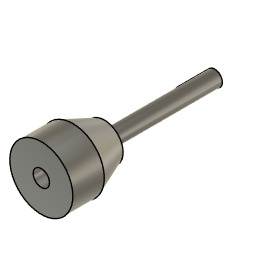
Motor_wheel_holder (Autodesk Fusion 360 archive; units mm, degrees)
design "Shaft"
Autodesk Fusion 360 part; units mm, degrees
sketch "Sketch1" plane through (0, 0, 0) normal (1, 0, 0) x (0, 1, 0)
  line L0 (0, 0) -> (55, 0) construction
  line L1 (55, 0) -> (55, 2.45)
  line L2 (20, 2.45) -> (20, 5.95)
  line L3 (12, 0) -> (9.8183, 2.6)
  line L4 (9.8183, 2.6) -> (0, 2.6)
  line L5 (12, 0) -> (55, 0)
  line L6 (0, 10) -> (0, 2.6)
  line L7 (20, 2.45) -> (55, 2.45)
  line L8 (0, 10) -> (10, 9.9769)
  line L9 (10, 9.9769) -> (20, 5.95)
  dimension "d1" = 2.45
  dimension "d3" = 50
  dimension "d4" = 12
  dimension "d5" = 20
  dimension "d7" = 2.6
  dimension "d8" = 55
  dimension "d18" = 10
  dimension "d19" = 10
  dimension "d20" = 158.199
  dimension "d21" = 3.5
  constraint coincident L0.start origin
  constraint horizontal L0
  constraint perpendicular L0 L1
  constraint coincident L0 L3.start
  constraint parallel L0 L4
  constraint perpendicular L4 L6
  constraint coincident L0.start L6
  constraint perpendicular L1 L7
  measures "d1" distance of L0.end L1.end
  measures "d3" angle of L0 L3
  measures "d4" distance of L3.start L6
  measures "d5" distance of L2 L6
  measures "d7" distance of L0.start L4
  measures "d8" distance of L1 L4.end
  measures "d18" distance of L0.start L8
  measures "d19" distance of L8.end L6.start
  measures "d20" angle of L8 L9
  measures "d21" distance of L2.end L7
revolve "Revolve1" add sketch "Sketch1" angle 360 about axis through (0, 0, 0) along (0, 1, 0)
ref_plane "WorkPlane1" through (-2.45, 48.8519, 0) normal (-1, 0, 0) x (0, 0, -1)
sketch "Sketch2" plane through (-2.45, 0, 0) normal (-1, 0, 0) x (0, -1, 0)
  line L0 (-55, -5) -> (-45, -5)
  line L1 (-45, -5) -> (-45, 5)
  line L2 (-45, 5) -> (-55, 5)
  line L3 (-55, 5) -> (-55, -5)
  constraint horizontal L0
  constraint vertical L1
  constraint horizontal L2
  constraint vertical L3
extrude "Extrude1" cut sketch "Sketch2" against normal blind 0.5
ref_plane "WorkPlane2" through (-9.9885, 5, 0) normal (-0.999997, 0.002314, 0) x (0, 0, -1)
sketch "Sketch3" plane through (-10, 0.0231, 0) normal (-0.999997, 0.002314, 0) x (-0.002314, -0.999997, 0)
  point P0 (-5, 0)
  dimension "d22" = 5
  measures "d22" distance of origin P0
hole "Hole1" at (-9.9884, 5.0231, 0) direction (0.999997, -0.002314, 0) diameter 4 depth 10 tip angle 118

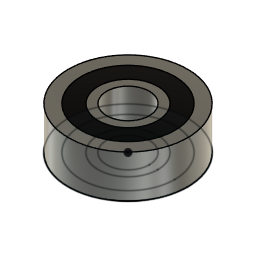
design "Bearing"
Autodesk Fusion 360 part; units mm, degrees
sketch "Sketch1" plane through (0, 0, 0) normal (0, 0, 1) x (1, 0, 0)
  circle A0 centre (0, 0) radius 7
  circle A1 centre (0, 0) radius 2.5
  circle A2 centre (0, 0) radius 3.5
  circle A3 centre (0, 0) radius 5.5
  dimension "d1" = 14
  dimension "d2" = 5
  dimension "d3" = 7
  dimension "d4" = 11
  constraint coincident A0.centre A1.centre
  constraint concentric A1 A2
  constraint concentric A2 A3
  measures "d1" diameter of A0
  measures "d2" diameter of A1
  measures "d3" diameter of A2
  measures "d4" diameter of A3
extrude "Extrude1" add sketch "Sketch1" along normal blind 5 contours A0 makes body 1
extrude "Extrude2" add sketch "Sketch1" along normal blind 5 separate body contours A3 makes body 2
extrude "Extrude3" add sketch "Sketch1" along normal blind 5 separate body contours A2 makes body 3
